Autodesk Inventor part; units mm, degrees
(part 2 of 3)
  line L933 (14.4439, 13.3712) -> (14.4659, 13.289)
  line L934 (14.4659, 13.289) -> (14.4484, 13.2234)
  line L935 (14.2154, 13.3626) -> (14.2397, 13.4369)
  line L936 (14.2397, 13.4369) -> (14.298, 13.5058)
  line L937 (14.298, 13.5058) -> (14.3807, 13.5279)
  line L938 (14.3807, 13.5279) -> (14.4634, 13.5058)
  line L939 (14.4634, 13.5058) -> (14.5239, 13.4453)
  line L940 (14.5239, 13.4453) -> (14.546, 13.3626)
  line L941 (14.546, 13.3626) -> (14.5239, 13.2799)
  line L942 (14.5239, 13.2799) -> (14.4484, 13.2234)
  line L943 (14.4484, 13.2234) -> (14.3807, 13.1972)
  line L944 (14.3807, 13.1972) -> (14.298, 13.2194)
  line L945 (14.298, 13.2194) -> (14.2375, 13.2799)
  line L946 (14.2375, 13.2799) -> (14.2154, 13.3626)
  line L947 (14.8734, 11.6652) -> (14.9343, 11.6816)
  line L948 (14.9343, 11.6816) -> (15.0165, 11.6595)
  line L949 (15.0165, 11.6595) -> (15.0767, 11.5993)
  line L950 (15.0767, 11.5993) -> (15.0987, 11.5171)
  line L951 (15.0987, 11.5171) -> (15.0767, 11.4349)
  line L952 (14.8517, 11.5809) -> (14.8734, 11.6652)
  line L953 (14.8734, 11.6652) -> (14.9343, 11.7241)
  line L954 (14.9343, 11.7241) -> (15.017, 11.7463)
  line L955 (15.017, 11.7463) -> (15.0997, 11.7241)
  line L956 (15.0997, 11.7241) -> (15.1602, 11.6636)
  line L957 (15.1602, 11.6636) -> (15.1823, 11.5809)
  line L958 (15.1823, 11.5809) -> (15.1602, 11.4982)
  line L959 (15.1602, 11.4982) -> (15.0997, 11.4377)
  line L960 (15.017, 11.4156) -> (14.9343, 11.4377)
  line L961 (14.9343, 11.4377) -> (14.8738, 11.4982)
  line L962 (14.8738, 11.4982) -> (14.8517, 11.5809)
  line L963 (14.8702, 9.3863) -> (14.9343, 9.4034)
  line L964 (14.9343, 9.4034) -> (15.0165, 9.3814)
  line L965 (15.0767, 9.1568) -> (15.0309, 9.111)
  line L966 (15.0165, 9.3814) -> (15.0767, 9.3212)
  line L967 (15.0767, 9.3212) -> (15.0987, 9.239)
  line L968 (15.0987, 9.239) -> (15.0767, 9.1568)
  line L969 (14.8517, 9.2902) -> (14.8702, 9.3863)
  line L970 (14.8702, 9.3863) -> (14.9343, 9.4334)
  line L971 (14.9343, 9.4334) -> (15.017, 9.4555)
  line L972 (15.017, 9.4555) -> (15.0997, 9.4334)
  line L973 (15.0997, 9.4334) -> (15.1602, 9.3729)
  line L974 (15.1602, 9.3729) -> (15.1823, 9.2902)
  line L975 (15.1823, 9.2902) -> (15.1602, 9.2075)
  line L976 (15.1602, 9.2075) -> (15.0997, 9.147)
  line L977 (15.0309, 9.111) -> (14.9343, 9.147)
  line L978 (14.9343, 9.147) -> (14.8738, 9.2075)
  line L979 (14.8738, 9.2075) -> (14.8517, 9.2902)
  line L980 (-2.5471, 11.8525) -> (-2.4869, 11.9127)
  line L981 (-2.5612, 11.9181) -> (-2.5007, 11.9786)
  line L982 (-2.1959, 13.1783) -> (-2.1357, 13.1181)
  line L983 (-2.2081, 13.2513) -> (-2.1475, 13.1907)
  line L984 (6.4547, 14.3394) -> (6.5369, 14.3173)
  line L985 (-16.6714, -15.6533) -> (-16.535, -15.1443)
  line L986 (-3.4172, 17.7096) -> (-3.0466, 17.339)
  line L987 (17.2697, -14.7625) -> (17.2918, -14.6798)
  line L988 (8.953, 17.2918) -> (8.8925, 17.3523)
  line L989 (8.8925, 17.3523) -> (8.8703, 17.435)
  line L990 (-2.3603, 13.1783) -> (-2.2781, 13.2003)
  line L991 (-2.3734, 13.2513) -> (-2.2907, 13.2734)
  line L992 (-4.4542, 16.0442) -> (-4.8268, 16.4169)
  line L993 (-2.1357, 13.1181) -> (-2.1475, 13.0254)
  line L994 (-2.2081, 12.9649) -> (-2.2907, 12.9427)
  line L995 (-2.4205, 13.1181) -> (-2.3603, 13.1783)
  line L996 (-2.4339, 13.1907) -> (-2.3734, 13.2513)
  line L997 (8.8925, 17.5177) -> (8.953, 17.5782)
  line L998 (8.9181, 14.1749) -> (8.9859, 13.9218)
  line L999 (16.0797, 11.6922) -> (16.0192, 11.7528)
  line L1000 (8.9859, 13.9218) -> (8.9277, 13.7046)
  line L1001 (8.4796, 14.4281) -> (8.7328, 14.3602)
  line L1002 (-2.1475, 13.1907) -> (-2.1357, 13.1181)
  line L1003 (-2.3067, 16.8433) -> (-2.3288, 16.9259)
  line L1004 (1.5431, 16.4996) -> (1.5652, 16.4169)
  line L1005 (8.2721, 14.4398) -> (8.5266, 14.508)
  line L1006 (8.0858, 14.2534) -> (8.2721, 14.4398)
  line L1007 (8.7811, 14.4398) -> (8.9675, 14.2534)
  line L1008 (16.0192, 11.7528) -> (15.997, 11.8354)
  line L1009 (8.5266, 14.508) -> (8.7811, 14.4398)
  line L1010 (-3.0634, 16.4169) -> (-3.4361, 16.0442)
  line L1011 (1.3999, 16.2516) -> (1.3172, 16.2737)
  line L1012 (-2.1475, 13.0254) -> (-2.2081, 12.9649)
  line L1013 (8.2265, 14.3602) -> (8.4796, 14.4281)
  line L1014 (8.0733, 14.207) -> (8.2265, 14.3602)
  line L1015 (9.0681, 17.4814) -> (9.1283, 17.4212)
  line L1016 (9.1183, 17.5782) -> (9.1788, 17.5177)
  line L1017 (8.7328, 14.3602) -> (8.9181, 14.1749)
  line L1018 (-3.4361, 16.0442) -> (-3.9451, 15.9078)
  line L1019 (-13.558, 10.4603) -> (-13.4978, 10.5205)
  line L1020 (8.9675, 14.2534) -> (9.0357, 13.9989)
  line L1021 (9.0357, 13.9989) -> (8.9675, 13.7444)
  line L1022 (8.7811, 13.5581) -> (8.5266, 13.4899)
  line L1023 (-14.8006, 2.418) -> (-14.7784, 2.5007)
  line L1024 (-3.9451, 15.9078) -> (-4.4542, 16.0442)
  line L1025 (8.5266, 13.4899) -> (8.2721, 13.5581)
  line L1026 (16.0192, 11.9181) -> (16.0797, 11.9786)
  line L1027 (1.4826, 16.2737) -> (1.3999, 16.2516)
  line L1028 (8.2721, 13.5581) -> (8.0858, 13.7444)
  line L1029 (1.4826, 16.5601) -> (1.5431, 16.4996)
  line L1030 (8.0858, 13.7444) -> (8.0176, 13.9989)
  line L1031 (8.9037, 17.4814) -> (8.9859, 17.5034)
  line L1032 (8.953, 17.5782) -> (9.0357, 17.6003)
  line L1033 (-2.2781, 13.2003) -> (-2.1959, 13.1783)
  line L1034 (-2.2907, 13.2734) -> (-2.2081, 13.2513)
  line L1035 (9.0357, 17.6003) -> (9.1183, 17.5782)
  line L1036 (16.2158, 11.8525) -> (16.2378, 11.7703)
  line L1037 (-4.9359, 16.8327) -> (-4.8003, 17.339)
  line L1038 (-3.9234, 17.8452) -> (-3.4172, 17.7096)
  line L1039 (-4.4297, 17.7096) -> (-3.9234, 17.8452)
  line L1040 (-4.8003, 17.339) -> (-4.4297, 17.7096)
  line L1041 (1.1391, 5.8597) -> (1.2213, 5.8377)
  line L1042 (1.0568, 5.8377) -> (1.1391, 5.8597)
  line L1043 (9.1503, 17.339) -> (9.1183, 17.2918)
  line L1044 (8.9859, 17.5034) -> (9.0681, 17.4814)
  line L1045 (8.8703, 17.435) -> (8.9037, 17.4814)
  line L1046 (-10.6691, 13.0359) -> (-10.647, 13.1181)
  line L1047 (-10.6497, 12.9637) -> (-10.6691, 13.0359)
  line L1048 (-10.5046, 13.2003) -> (-10.4229, 13.1784)
  line L1049 (-10.5868, 13.1783) -> (-10.5046, 13.2003)
  line L1050 (-10.647, 13.1181) -> (-10.5868, 13.1783)
  line L1051 (1.5346, 16.4087) -> (1.5538, 16.3371)
  line L1052 (1.4744, 16.4689) -> (1.5346, 16.4087)
  line L1053 (1.3922, 16.4909) -> (1.4744, 16.4689)
  line L1054 (1.31, 16.4689) -> (1.3922, 16.4909)
  line L1055 (1.2498, 16.4087) -> (1.31, 16.4689)
  line L1056 (-11.6816, 14.3015) -> (-11.6595, 14.3837)
  line L1057 (-11.6644, 14.2373) -> (-11.6816, 14.3015)
  line L1058 (-11.5171, 14.4659) -> (-11.4424, 14.4459)
  line L1059 (-11.5993, 14.4439) -> (-11.5171, 14.4659)
  line L1060 (-11.6595, 14.3837) -> (-11.5993, 14.4439)
  line L1061 (-13.58, 12.4031) -> (-13.558, 12.4853)
  line L1062 (-13.5609, 12.3317) -> (-13.58, 12.4031)
  line L1063 (-13.4156, 12.5675) -> (-13.348, 12.5494)
  line L1064 (-13.4978, 12.5455) -> (-13.4156, 12.5675)
  line L1065 (-13.558, 12.4853) -> (-13.4978, 12.5455)
  line L1066 (-14.5925, 11.3906) -> (-14.5705, 11.4728)
  line L1067 (-14.5723, 11.3154) -> (-14.5925, 11.3906)
  line L1068 (-14.4281, 11.555) -> (-14.3643, 11.5379)
  line L1069 (-14.5103, 11.533) -> (-14.4281, 11.555)
  line L1070 (-14.5705, 11.4728) -> (-14.5103, 11.533)
  line L1071 (-8.391, 17.339) -> (-8.3689, 17.4212)
  line L1072 (-8.1443, 17.4814) -> (-8.1023, 17.4394)
  line L1073 (-8.2265, 17.5034) -> (-8.1443, 17.4814)
  line L1074 (-8.3087, 17.4814) -> (-8.2265, 17.5034)
  line L1075 (-8.3689, 17.4212) -> (-8.3087, 17.4814)
  line L1076 (-7.1232, 17.3471) -> (-7.1033, 17.4212)
  line L1077 (-6.8787, 17.4814) -> (-6.8332, 17.4359)
  line L1078 (-6.9609, 17.5034) -> (-6.8787, 17.4814)
  line L1079 (-7.0431, 17.4814) -> (-6.9609, 17.5034)
  line L1080 (-7.1033, 17.4212) -> (-7.0431, 17.4814)
  line L1081 (-17.5034, 5.9484) -> (-17.4814, 6.0306)
  line L1082 (-17.4814, 5.8662) -> (-17.5034, 5.9484)
  line L1083 (-17.4331, 5.8179) -> (-17.4814, 5.8662)
  line L1084 (-17.4212, 6.0908) -> (-17.3485, 6.1103)
  line L1085 (-17.4814, 6.0306) -> (-17.4212, 6.0908)
  line L1086 (-17.5034, 0.8859) -> (-17.4814, 0.9681)
  line L1087 (-17.4814, 0.8037) -> (-17.5034, 0.8859)
  line L1088 (-17.4212, 0.7435) -> (-17.4814, 0.8037)
  line L1089 (-17.3944, 0.7364) -> (-17.4212, 0.7435)
  line L1090 (-17.4212, 1.0283) -> (-17.3555, 1.0459)
  line L1091 (-17.4814, 0.9681) -> (-17.4212, 1.0283)
  line L1092 (-14.3394, -4.4297) -> (-14.3173, -4.3474)
  line L1093 (-14.3173, -4.5119) -> (-14.3394, -4.4297)
  line L1094 (-14.2571, -4.5721) -> (-14.3173, -4.5119)
  line L1095 (-14.1749, -4.5941) -> (-14.2571, -4.5721)
  line L1096 (-14.3173, -4.3474) -> (-14.2571, -4.2873)
  line L1097 (-17.3768, -10.5046) -> (-17.3548, -10.4224)
  line L1098 (-17.3548, -10.5868) -> (-17.3768, -10.5046)
  line L1099 (-17.2946, -10.647) -> (-17.3548, -10.5868)
  line L1100 (-17.2124, -10.6691) -> (-17.2946, -10.647)
  line L1101 (-17.1619, -10.6555) -> (-17.2124, -10.6691)
  line L1102 (-17.3548, -10.4224) -> (-17.3188, -10.3864)
  line L1103 (-14.4659, -12.5296) -> (-14.4473, -12.4601)
  line L1104 (-14.4439, -12.6118) -> (-14.4659, -12.5296)
  line L1105 (-14.3837, -12.672) -> (-14.4439, -12.6118)
  line L1106 (-14.3015, -12.6941) -> (-14.3837, -12.672)
  line L1107 (-14.2387, -12.6772) -> (-14.3015, -12.6941)
  line L1108 (-15.7315, -6.9609) -> (-15.7095, -6.8787)
  line L1109 (-15.7095, -7.0431) -> (-15.7315, -6.9609)
  line L1110 (-15.6493, -7.1033) -> (-15.7095, -7.0431)
  line L1111 (-15.5671, -7.1253) -> (-15.6493, -7.1033)
  line L1112 (-15.7095, -6.8787) -> (-15.6591, -6.8283)
  line L1113 (-14.4659, -10.7578) -> (-14.4448, -10.6791)
  line L1114 (-14.4439, -10.84) -> (-14.4659, -10.7578)
  line L1115 (-14.3837, -10.9002) -> (-14.4439, -10.84)
  line L1116 (-14.3015, -10.9222) -> (-14.3837, -10.9002)
  line L1117 (-14.2362, -10.9047) -> (-14.3015, -10.9222)
  line L1118 (-16.9972, -12.0234) -> (-16.9751, -11.9412)
  line L1119 (-16.9751, -12.1056) -> (-16.9972, -12.0234)
  line L1120 (-16.9149, -12.1658) -> (-16.9751, -12.1056)
  line L1121 (-16.8327, -12.1878) -> (-16.9149, -12.1658)
  line L1122 (-16.7823, -12.1743) -> (-16.8327, -12.1878)
  line L1123 (-17.2503, -13.5421) -> (-17.2296, -13.4649)
  line L1124 (-17.2283, -13.6243) -> (-17.2503, -13.5421)
  line L1125 (-17.1681, -13.6845) -> (-17.2283, -13.6243)
  line L1126 (-17.0859, -13.7065) -> (-17.1681, -13.6845)
  line L1127 (-17.0388, -13.694) -> (-17.0859, -13.7065)
  line L1128 (-11.1753, -15.314) -> (-11.1593, -15.2543)
  line L1129 (-11.1533, -15.3962) -> (-11.1753, -15.314)
  line L1130 (-11.0931, -15.4564) -> (-11.1533, -15.3962)
  line L1131 (-11.0109, -15.4784) -> (-11.0931, -15.4564)
  line L1132 (-10.9287, -15.4564) -> (-11.0109, -15.4784)
  line L1133 (-8.8972, -17.339) -> (-8.8832, -17.2866)
  line L1134 (-8.8752, -17.4212) -> (-8.8972, -17.339)
  line L1135 (-8.815, -17.4814) -> (-8.8752, -17.4212)
  line L1136 (-8.7328, -17.5034) -> (-8.815, -17.4814)
  line L1137 (-8.6506, -17.4814) -> (-8.7328, -17.5034)
  line L1138 (-8.61, -17.4408) -> (-8.6506, -17.4814)
  line L1139 (-6.5971, -17.4212) -> (-6.6167, -17.3478)
  line L1140 (-6.5369, -17.4814) -> (-6.5971, -17.4212)
  line L1141 (-6.4547, -17.5034) -> (-6.5369, -17.4814)
  line L1142 (-6.3724, -17.4814) -> (-6.4547, -17.5034)
  line L1143 (-6.3256, -17.4345) -> (-6.3724, -17.4814)
  line L1144 (-0.0158, -17.4212) -> (-0.0331, -17.3569)
  line L1145 (0.0443, -17.4814) -> (-0.0158, -17.4212)
  line L1146 (0.1266, -17.5034) -> (0.0443, -17.4814)
  line L1147 (0.2088, -17.4814) -> (0.1266, -17.5034)
  line L1148 (0.2863, -17.3566) -> (0.269, -17.4212)
  line L1149 (5.8662, -15.7095) -> (5.813, -15.6563)
  line L1150 (5.9484, -15.7315) -> (5.8662, -15.7095)
  line L1151 (6.0306, -15.7095) -> (5.9484, -15.7315)
  line L1152 (6.0908, -15.6493) -> (6.0306, -15.7095)
  line L1153 (6.1127, -15.5675) -> (6.0908, -15.6493)
  line L1154 (8.9037, -14.9501) -> (8.8568, -14.9033)
  line L1155 (8.9859, -14.9722) -> (8.9037, -14.9501)
  line L1156 (9.0681, -14.9501) -> (8.9859, -14.9722)
  line L1157 (9.1283, -14.89) -> (9.0681, -14.9501)
  line L1158 (9.1503, -14.8077) -> (9.1283, -14.89)
  line L1159 (9.1329, -14.7427) -> (9.1503, -14.8077)
  line L1160 (11.7703, -14.9722) -> (11.6975, -14.9527)
  line L1161 (11.8525, -14.9501) -> (11.7703, -14.9722)
  line L1162 (11.9127, -14.89) -> (11.8525, -14.9501)
  line L1163 (11.9347, -14.8077) -> (11.9127, -14.89)
  line L1164 (11.9183, -14.7465) -> (11.9347, -14.8077)
  line L1165 (13.5421, -15.9847) -> (13.467, -15.9645)
  line L1166 (13.6243, -15.9626) -> (13.5421, -15.9847)
  line L1167 (13.6845, -15.9024) -> (13.6243, -15.9626)
  line L1168 (13.7065, -15.8202) -> (13.6845, -15.9024)
  line L1169 (13.6922, -15.7667) -> (13.7065, -15.8202)
  line L1170 (15.0609, -17.3768) -> (14.9925, -17.3585)
  line L1171 (15.1431, -17.3548) -> (15.0609, -17.3768)
  line L1172 (15.2033, -17.2946) -> (15.1431, -17.3548)
  line L1173 (15.2253, -17.2124) -> (15.2033, -17.2946)
  line L1174 (15.2134, -17.1682) -> (15.2253, -17.2124)
  line L1175 (17.339, -14.8456) -> (17.2949, -14.8338)
  line L1176 (17.4212, -14.8236) -> (17.339, -14.8456)
  line L1177 (17.4814, -14.7634) -> (17.4212, -14.8236)
  line L1178 (17.5034, -14.6812) -> (17.4814, -14.7634)
  line L1179 (17.4844, -14.6104) -> (17.5034, -14.6812)
  line L1180 (15.5671, -13.4534) -> (15.5119, -13.4386)
  line L1181 (15.6493, -13.4314) -> (15.5671, -13.4534)
  line L1182 (15.7095, -13.3712) -> (15.6493, -13.4314)
  line L1183 (15.7315, -13.289) -> (15.7095, -13.3712)
  line L1184 (15.7111, -13.2127) -> (15.7315, -13.289)
  line L1185 (17.4814, 9.1568) -> (17.4422, 9.1176)
  line L1186 (17.5034, 9.239) -> (17.4814, 9.1568)
  line L1187 (17.4814, 9.3212) -> (17.5034, 9.239)
  line L1188 (17.4212, 9.3814) -> (17.4814, 9.3212)
  line L1189 (17.339, 9.4034) -> (17.4212, 9.3814)
  line L1190 (17.2873, 9.3896) -> (17.339, 9.4034)
  line L1191 (17.4814, 11.4349) -> (17.4485, 11.4021)
  line L1192 (17.5034, 11.5171) -> (17.4814, 11.4349)
  line L1193 (17.4814, 11.5993) -> (17.5034, 11.5171)
  line L1194 (17.4212, 11.6595) -> (17.4814, 11.5993)
  line L1195 (17.339, 11.6816) -> (17.4212, 11.6595)
  line L1196 (17.2905, 11.6686) -> (17.339, 11.6816)
  line L1197 (17.2503, 12.7827) -> (17.2284, 12.701)
  line L1198 (17.2283, 12.865) -> (17.2503, 12.7827)
  line L1199 (17.1681, 12.9251) -> (17.2283, 12.865)
  line L1200 (17.0859, 12.9472) -> (17.1681, 12.9251)
  line L1201 (17.0373, 12.9362) -> (17.0859, 12.9472)
  line L1202 (15.9847, 13.0359) -> (15.9637, 12.9577)
  line L1203 (14.2128, 17.339) -> (14.2007, 17.294)
  line L1204 (14.1908, 17.4212) -> (14.2128, 17.339)
  line L1205 (14.1306, 17.4814) -> (14.1908, 17.4212)
  line L1206 (14.0484, 17.5034) -> (14.1306, 17.4814)
  line L1207 (13.9738, 17.4834) -> (14.0484, 17.5034)
  line L1208 (12.9472, 17.339) -> (12.9347, 17.2922)
  line L1209 (12.9251, 17.4212) -> (12.9472, 17.339)
  line L1210 (12.865, 17.4814) -> (12.9251, 17.4212)
  line L1211 (12.7827, 17.5034) -> (12.865, 17.4814)
  line L1212 (12.7006, 17.4814) -> (12.7827, 17.5034)
  line L1213 (10.9222, 17.339) -> (10.9089, 17.2894)
  line L1214 (16.2378, 11.7703) -> (16.2158, 11.688)
  line L1215 (16.1556, 11.9127) -> (16.2158, 11.8525)
  line L1216 (16.0192, 11.9181) -> (16.0734, 11.9347)
  line L1217 (6.5971, 14.2571) -> (6.6191, 14.1749)
  line L1218 (6.5369, 14.3173) -> (6.5971, 14.2571)
  line L1219 (5.5846, 14.004) -> (5.6155, 13.9162)
  line L1220 (5.5244, 14.0642) -> (5.5846, 14.004)
  line L1221 (5.4422, 14.0862) -> (5.5244, 14.0642)
  line L1222 (5.3599, 14.0642) -> (5.4422, 14.0862)
  line L1223 (-5.8662, 16.4689) -> (-5.8151, 16.4178)
  line L1224 (-5.9484, 16.4909) -> (-5.8662, 16.4689)
  line L1225 (-6.0306, 16.4689) -> (-5.9484, 16.4909)
  line L1226 (-6.0908, 16.4087) -> (-6.0306, 16.4689)
  line L1227 (-6.1128, 15.0609) -> (-6.0908, 15.1431)
  line L1228 (-5.8662, 15.2033) -> (-5.8116, 15.1487)
  line L1229 (-5.9484, 15.2253) -> (-5.8662, 15.2033)
  line L1230 (-6.0306, 15.2033) -> (-5.9484, 15.2253)
  line L1231 (-6.0908, 15.1431) -> (-6.0306, 15.2033)
  line L1232 (-4.3409, 15.0611) -> (-4.3189, 15.1431)
  line L1233 (-4.0943, 15.2033) -> (-4.0348, 15.1438)
  line L1234 (-4.1765, 15.2253) -> (-4.0943, 15.2033)
  line L1235 (-4.2588, 15.2033) -> (-4.1765, 15.2253)
  line L1236 (-4.3189, 15.1431) -> (-4.2588, 15.2033)
  line L1237 (-12.4031, 11.555) -> (-12.3286, 11.5363)
  line L1238 (-12.4853, 11.533) -> (-12.4031, 11.555)
  line L1239 (-15.4784, 10.5046) -> (-15.4564, 10.5868)
  line L1240 (-15.4564, 10.4224) -> (-15.4784, 10.5046)
  line L1241 (-15.314, 10.6691) -> (-15.2536, 10.6529)
  line L1242 (-15.3962, 10.647) -> (-15.314, 10.6691)
  line L1243 (-15.4564, 10.5868) -> (-15.3962, 10.647)
  line L1244 (-2.3067, 16.8433) -> (-2.294, 16.9149)
  line L1245 (-2.0693, 16.9751) -> (-2.0092, 16.9149)
  line L1246 (-2.1516, 16.9972) -> (-2.0693, 16.9751)
  line L1247 (-2.2338, 16.9751) -> (-2.1516, 16.9972)
  line L1248 (-2.294, 16.9149) -> (-2.2338, 16.9751)
  line L1249 (-13.58, 10.3781) -> (-13.558, 10.4603)
  line L1250 (-13.5581, 10.2962) -> (-13.58, 10.3781)
  line L1251 (-13.4978, 10.5205) -> (-13.4156, 10.5425)
  line L1252 (-14.2128, 3.6703) -> (-14.1908, 3.7525)
  line L1253 (-14.1908, 3.5881) -> (-14.2128, 3.6703)
  line L1254 (-14.1306, 3.5279) -> (-14.1908, 3.5881)
  line L1255 (-14.1306, 3.8127) -> (-14.0484, 3.8347)
  line L1256 (-14.1908, 3.7525) -> (-14.1306, 3.8127)
  line L1257 (-17.4814, -0.8416) -> (-17.5034, -0.7594)
  line L1258 (-17.4212, -0.9018) -> (-17.4814, -0.8416)
  line L1259 (-17.3557, -0.9193) -> (-17.4212, -0.9018)
  line L1260 (-16.2378, -0.6328) -> (-16.2158, -0.5506)
  line L1261 (-16.2158, -0.715) -> (-16.2378, -0.6328)
  line L1262 (-16.1556, -0.7752) -> (-16.2158, -0.715)
  line L1263 (-16.0837, -0.7945) -> (-16.1556, -0.7752)
  line L1264 (-16.2158, -0.5506) -> (-16.1556, -0.4904)
  line L1265 (-15.0987, -5.6953) -> (-15.0767, -5.6131)
  line L1266 (-15.0767, -5.7775) -> (-15.0987, -5.6953)
  line L1267 (-15.0165, -5.8377) -> (-15.0767, -5.7775)
  line L1268 (-14.9343, -5.8597) -> (-15.0165, -5.8377)
  line L1269 (-15.0767, -5.6131) -> (-15.0211, -5.5574)
  line L1270 (-13.7065, -5.9484) -> (-13.6845, -5.8662)
  line L1271 (-13.6845, -6.0306) -> (-13.7065, -5.9484)
  line L1272 (-13.6243, -6.0908) -> (-13.6845, -6.0306)
  line L1273 (-13.5421, -6.1128) -> (-13.6243, -6.0908)
  line L1274 (-13.6845, -5.8662) -> (-13.6257, -5.8074)
  line L1275 (-14.2128, -7.9734) -> (-14.1908, -7.8912)
  line L1276 (-14.1908, -8.0556) -> (-14.2128, -7.9734)
  line L1277 (-14.1306, -8.1158) -> (-14.1908, -8.0556)
  line L1278 (-14.0484, -8.1378) -> (-14.1306, -8.1158)
  line L1279 (-13.978, -8.119) -> (-14.0484, -8.1378)
  line L1280 (-14.1908, -7.8912) -> (-14.139, -7.8394)
  line L1281 (-12.4409, -12.2765) -> (-12.4212, -12.2029)
  line L1282 (-12.4189, -12.3587) -> (-12.4409, -12.2765)
  line L1283 (-12.3587, -12.4189) -> (-12.4189, -12.3587)
  line L1284 (-12.2765, -12.4409) -> (-12.3587, -12.4189)
  line L1285 (-12.2029, -12.4212) -> (-12.2765, -12.4409)
  line L1286 (-8.7706, -13.7952) -> (-8.7517, -13.7244)
  line L1287 (-8.7486, -13.8775) -> (-8.7706, -13.7952)
  line L1288 (-8.6884, -13.9376) -> (-8.7486, -13.8775)
  line L1289 (-8.6062, -13.9597) -> (-8.6884, -13.9376)
  line L1290 (-8.524, -13.9376) -> (-8.6062, -13.9597)
  line L1291 (-8.4997, -13.9134) -> (-8.524, -13.9376)
  line L1292 (0.8037, -15.4564) -> (0.7435, -15.3962)
  line L1293 (0.8859, -15.4784) -> (0.8037, -15.4564)
  line L1294 (0.9681, -15.4564) -> (0.8859, -15.4784)
  line L1295 (1.0283, -15.3962) -> (0.9681, -15.4564)
  line L1296 (1.0487, -15.3201) -> (1.0283, -15.3962)
  line L1297 (13.558, -13.4978) -> (13.4978, -13.558)
  line L1298 (13.58, -13.4156) -> (13.558, -13.4978)
  line L1299 (13.5623, -13.3494) -> (13.58, -13.4156)
  line L1300 (13.3269, 10.5046) -> (13.305, 10.4231)
  line L1301 (13.3048, 10.5868) -> (13.3269, 10.5046)
  line L1302 (13.2446, 10.647) -> (13.3048, 10.5868)
  line L1303 (13.1624, 10.6691) -> (13.2446, 10.647)
  line L1304 (13.0909, 10.6499) -> (13.1624, 10.6691)
  line L1305 (11.1832, 12.9362) -> (11.264, 12.9472)
  line L1306 (-17.5034, 4.05) -> (-17.4814, 4.1322)
  line L1307 (-17.4814, 3.9678) -> (-17.5034, 4.05)
  line L1308 (-17.4278, 3.9142) -> (-17.4814, 3.9678)
  line L1309 (-17.4212, 4.1924) -> (-17.3511, 4.2112)
  line L1310 (-17.4814, 4.1322) -> (-17.4212, 4.1924)
  line L1311 (-17.5034, 2.5312) -> (-17.4814, 2.6135)
  line L1312 (-17.4236, 2.3913) -> (-17.4814, 2.449)
  line L1313 (-17.4212, 2.6736) -> (-17.3532, 2.6918)
  line L1314 (-17.4814, 2.6135) -> (-17.4212, 2.6736)
  line L1315 (-5.2049, -0.0822) -> (-5.2269, 0)
  line L1316 (-5.1447, -0.1424) -> (-5.2049, -0.0822)
  line L1317 (1.5346, 12.2322) -> (1.5566, 12.1499)
  line L1318 (1.4744, 12.2923) -> (1.5346, 12.2322)
  line L1319 (1.3922, 12.3144) -> (1.4744, 12.2923)
  line L1320 (1.31, 12.2923) -> (1.3922, 12.3144)
  line L1321 (1.2498, 12.2322) -> (1.31, 12.2923)
  line L1322 (-3.455, 12.6562) -> (-3.433, 12.7384)
  line L1323 (-3.2084, 12.7986) -> (-3.1482, 12.7384)
  line L1324 (-3.2906, 12.8206) -> (-3.2084, 12.7986)
  line L1325 (-3.3728, 12.7986) -> (-3.2906, 12.8206)
  line L1326 (-3.433, 12.7384) -> (-3.3728, 12.7986)
  line L1327 (-2.5691, 11.7703) -> (-2.5471, 11.8525)
  line L1328 (-2.3225, 11.9127) -> (-2.2623, 11.8525)
  line L1329 (-2.4047, 11.9347) -> (-2.3225, 11.9127)
  line L1330 (-2.4869, 11.9127) -> (-2.4047, 11.9347)
  line L1331 (-1.3035, 13.0359) -> (-1.2815, 13.1181)
  line L1332 (-1.0568, 13.1783) -> (-0.9967, 13.1181)
  line L1333 (-1.1391, 13.2003) -> (-1.0568, 13.1783)
  line L1334 (-1.2213, 13.1783) -> (-1.1391, 13.2003)
  line L1335 (-1.2815, 13.1181) -> (-1.2213, 13.1783)
  line L1336 (4.4455, 12.9915) -> (4.4675, 12.9093)
  line L1337 (4.3853, 13.0517) -> (4.4455, 12.9915)
  line L1338 (4.3031, 13.0737) -> (4.3853, 13.0517)
  line L1339 (4.2209, 13.0517) -> (4.3031, 13.0737)
  line L1340 (4.1607, 12.9915) -> (4.2209, 13.0517)
  line L1341 (-3.7525, -2.294) -> (-3.8127, -2.2338)
  line L1342 (1.4744, 8.622) -> (1.5346, 8.5619)
  line L1343 (1.3922, 8.6441) -> (1.4744, 8.622)
  line L1344 (1.31, 8.622) -> (1.3922, 8.6441)
  line L1345 (1.2498, 8.5619) -> (1.31, 8.622)
  line L1346 (15.0767, 4.6006) -> (15.0183, 4.5421)
  line L1347 (15.0987, 4.6828) -> (15.0767, 4.6006)
  line L1348 (15.0767, 4.765) -> (15.0987, 4.6828)
  line L1349 (15.0165, 4.8252) -> (15.0767, 4.765)
  line L1350 (14.9343, 4.8472) -> (15.0165, 4.8252)
  line L1351 (15.3962, -0.7752) -> (15.3161, -0.7795)
  line L1352 (15.4564, -0.715) -> (15.3962, -0.7752)
  line L1353 (15.4784, -0.6328) -> (15.4564, -0.715)
  line L1354 (15.4564, -0.5506) -> (15.4784, -0.6328)
  line L1355 (15.3988, -0.471) -> (15.4564, -0.5506)
  line L1356 (-13.4534, 2.1516) -> (-13.4314, 2.2338)
  line L1357 (-13.4314, 2.0693) -> (-13.4534, 2.1516)
  line L1358 (-13.3712, 2.0092) -> (-13.4314, 2.0693)
  line L1359 (-13.3712, 2.294) -> (-13.289, 2.316)
  line L1360 (-13.4314, 2.2338) -> (-13.3712, 2.294)
  line L1361 (-14.719, 2.4047) -> (-14.697, 2.4869)
  line L1362 (-14.697, 2.3225) -> (-14.719, 2.4047)
  line L1363 (-14.6368, 2.2623) -> (-14.697, 2.3225)
  line L1364 (-14.6368, 2.5471) -> (-14.5547, 2.5691)
  line L1365 (-14.697, 2.4869) -> (-14.6368, 2.5471)
  line L1366 (-11.1753, -2.1516) -> (-11.1533, -2.0693)
  line L1367 (-11.1533, -2.2338) -> (-11.1753, -2.1516)
  line L1368 (-11.0931, -2.294) -> (-11.1533, -2.2338)
  line L1369 (-11.0109, -2.316) -> (-11.0931, -2.294)
  line L1370 (-11.1533, -2.0693) -> (-11.0931, -2.0092)
  line L1371 (-16.9751, 7.0052) -> (-16.9972, 7.0875)
  line L1372 (-16.9286, 6.9587) -> (-16.9751, 7.0052)
  line L1373 (-16.9149, 7.2299) -> (-16.8381, 7.2505)
  line L1374 (-16.9751, 7.1697) -> (-16.9149, 7.2299)
  line L1375 (-7.9734, 7.7203) -> (-7.9395, 7.8468)
  line L1376 (-7.9395, 7.5937) -> (-7.9734, 7.7203)
  line L1377 (-7.7203, 7.9734) -> (-7.5937, 7.9395)
  line L1378 (-7.8468, 7.9395) -> (-7.7203, 7.9734)
  line L1379 (-7.9395, 7.8468) -> (-7.8468, 7.9395)
  line L1380 (7.9734, 7.7203) -> (7.9395, 7.5937)
  line L1381 (7.9395, 7.8468) -> (7.9734, 7.7203)
  line L1382 (7.8468, 7.9395) -> (7.9395, 7.8468)
  line L1383 (7.7203, 7.9734) -> (7.8468, 7.9395)
  line L1384 (7.5937, 7.9395) -> (7.7203, 7.9734)
  line L1385 (-7.9395, -7.8468) -> (-7.9734, -7.7203)
  line L1386 (-7.8468, -7.9395) -> (-7.9395, -7.8468)
  line L1387 (-7.5937, -7.9395) -> (-7.7203, -7.9734)
  line L1388 (7.7203, -7.9734) -> (7.5937, -7.9395)
  line L1389 (7.8468, -7.9395) -> (7.7203, -7.9734)
  line L1390 (7.9734, -7.7203) -> (7.9395, -7.8468)
  line L1391 (16.3056, 11.9181) -> (16.3277, 11.8354)
  line L1392 (-15.6533, -14.6352) -> (-15.1443, -14.7716)
  line L1393 (-15.1443, -14.7716) -> (-14.7716, -15.1443)
  line L1394 (-14.7716, -15.1443) -> (-14.6352, -15.6533)
  line L1395 (-14.6352, -15.6533) -> (-14.7716, -16.1624)
  line L1396 (-15.1443, -16.535) -> (-15.6533, -16.6714)
  line L1397 (-15.6533, -16.6714) -> (-16.1624, -16.535)
  line L1398 (-16.1624, -16.535) -> (-16.535, -16.1624)
  line L1399 (-16.535, -16.1624) -> (-16.6714, -15.6533)
  line L1400 (-4.9632, 16.9259) -> (-4.8268, 17.435)
  line L1401 (-4.8268, 17.435) -> (-4.4542, 17.8076)
  line L1402 (-4.4542, 17.8076) -> (-3.9451, 17.944)
  line L1403 (-3.9451, 17.944) -> (-3.4361, 17.8076)
  line L1404 (-3.4361, 17.8076) -> (-3.0634, 17.435)
  line L1405 (-2.927, 16.9259) -> (-3.0634, 16.4169)
  line L1406 (0.98, 5.7268) -> (1.0022, 5.8095)
  line L1407 (1.0627, 5.87) -> (1.1454, 5.8922)
  line L1408 (1.1454, 5.8922) -> (1.228, 5.87)
  line L1409 (1.228, 5.87) -> (1.2886, 5.8095)
  line L1410 (1.2886, 5.6442) -> (1.228, 5.5836)
  line L1411 (1.228, 5.5836) -> (1.1454, 5.5615)
  line L1412 (1.1454, 5.5615) -> (1.0627, 5.5836)
  line L1413 (1.0627, 5.5836) -> (1.0022, 5.6442)
  line L1414 (1.0022, 5.6442) -> (0.98, 5.7268)
  line L1415 (-2.2907, 12.9427) -> (-2.3734, 12.9649)
  line L1416 (-2.3734, 12.9649) -> (-2.4425, 13.0359)
  line L1417 (-2.4425, 13.0359) -> (-2.4561, 13.1081)
  line L1418 (9.201, 17.435) -> (9.1788, 17.3523)
  line L1419 (9.1183, 17.2918) -> (9.0357, 17.2697)
  line L1420 (11.6922, 17.5177) -> (11.7528, 17.5782)
  line L1421 (11.7528, 17.5782) -> (11.8354, 17.6003)
  line L1422 (11.8354, 17.6003) -> (11.9181, 17.5782)
  line L1423 (11.9181, 17.5782) -> (11.9786, 17.5177)
  line L1424 (11.9786, 17.5177) -> (12.0008, 17.435)
  line L1425 (12.0008, 17.435) -> (11.9786, 17.3523)
  line L1426 (11.9786, 17.3523) -> (11.9218, 17.2908)
  line L1427 (11.9218, 17.2908) -> (11.8354, 17.2697)
  line L1428 (11.8354, 17.2697) -> (11.7528, 17.2918)
  line L1429 (11.7528, 17.2918) -> (11.6922, 17.3523)
  line L1430 (11.6922, 17.3523) -> (11.6559, 17.4492)
  line L1431 (-10.7282, 13.1081) -> (-10.706, 13.1907)
  line L1432 (-10.706, 13.1907) -> (-10.6455, 13.2513)
  line L1433 (-10.6455, 13.2513) -> (-10.5628, 13.2734)
  line L1434 (-10.5628, 13.2734) -> (-10.4801, 13.2513)
  line L1435 (-10.4801, 13.2513) -> (-10.4229, 13.1784)
  line L1436 (-10.4229, 13.1784) -> (-10.3975, 13.1081)
  line L1437 (-10.3975, 13.1081) -> (-10.4196, 13.0254)
  line L1438 (-10.4196, 13.0254) -> (-10.4801, 12.9649)
  line L1439 (-10.4801, 12.9649) -> (-10.5628, 12.9427)
  line L1440 (-10.5628, 12.9427) -> (-10.6497, 12.9637)
  line L1441 (-10.6497, 12.9637) -> (-10.706, 13.0254)
  line L1442 (-10.706, 13.0254) -> (-10.7282, 13.1081)
  line L1443 (1.2498, 16.4087) -> (1.2567, 16.4996)
  line L1444 (1.3172, 16.5601) -> (1.3999, 16.5822)
  line L1445 (1.5652, 16.4169) -> (1.5538, 16.3371)
  line L1446 (1.5538, 16.3371) -> (1.4826, 16.2737)
  line L1447 (1.3172, 16.2737) -> (1.2567, 16.3342)
  line L1448 (1.2567, 16.3342) -> (1.2498, 16.4087)
  line L1449 (-11.7463, 14.3807) -> (-11.7241, 14.4634)
  line L1450 (-11.7241, 14.4634) -> (-11.6636, 14.5239)
  line L1451 (-11.6636, 14.5239) -> (-11.5809, 14.546)
  line L1452 (-11.5809, 14.546) -> (-11.4982, 14.5239)
  line L1453 (-11.4982, 14.5239) -> (-11.4424, 14.4459)
  line L1454 (-11.4424, 14.4459) -> (-11.4156, 14.3807)
  line L1455 (-11.4156, 14.3807) -> (-11.4377, 14.298)
  line L1456 (-11.4377, 14.298) -> (-11.4982, 14.2375)
  line L1457 (-11.4982, 14.2375) -> (-11.5809, 14.2154)
  line L1458 (-11.5809, 14.2154) -> (-11.6644, 14.2373)
  line L1459 (-11.6644, 14.2373) -> (-11.7241, 14.298)
  line L1460 (-11.7241, 14.298) -> (-11.7463, 14.3807)
  line L1461 (-13.6552, 12.4718) -> (-13.633, 12.5544)
  line L1462 (-13.633, 12.5544) -> (-13.5725, 12.6149)
  line L1463 (-13.5725, 12.6149) -> (-13.4899, 12.6371)
  line L1464 (-13.4899, 12.6371) -> (-13.4072, 12.6149)
  line L1465 (-13.4072, 12.6149) -> (-13.348, 12.5494)
  line L1466 (-13.348, 12.5494) -> (-13.3245, 12.4718)
  line L1467 (-13.3245, 12.4718) -> (-13.3467, 12.3891)
  line L1468 (-13.3467, 12.3891) -> (-13.4072, 12.3286)
  line L1469 (-13.4072, 12.3286) -> (-13.4899, 12.3064)
  line L1470 (-13.4899, 12.3064) -> (-13.5609, 12.3317)
  line L1471 (-13.5609, 12.3317) -> (-13.633, 12.3891)
  line L1472 (-13.633, 12.3891) -> (-13.6552, 12.4718)
  line L1473 (-14.6733, 11.4536) -> (-14.6511, 11.5363)
  line L1474 (-14.6511, 11.5363) -> (-14.5906, 11.5968)
  line L1475 (-14.5906, 11.5968) -> (-14.508, 11.619)
  line L1476 (-14.508, 11.619) -> (-14.4253, 11.5968)
  line L1477 (-14.4253, 11.5968) -> (-14.3643, 11.5379)
  line L1478 (-14.3643, 11.5379) -> (-14.3426, 11.4536)
  line L1479 (-14.3426, 11.4536) -> (-14.3648, 11.371)
  line L1480 (-14.3648, 11.371) -> (-14.4253, 11.3105)
  line L1481 (-14.4253, 11.3105) -> (-14.508, 11.2883)
  line L1482 (-14.508, 11.2883) -> (-14.5723, 11.3154)
  line L1483 (-14.5723, 11.3154) -> (-14.6511, 11.371)
  line L1484 (-14.6511, 11.371) -> (-14.6733, 11.4536)
  line L1485 (-8.4374, 17.435) -> (-8.4153, 17.5177)
  line L1486 (-8.4153, 17.5177) -> (-8.3547, 17.5782)
  line L1487 (-8.3547, 17.5782) -> (-8.2721, 17.6003)
  line L1488 (-8.2721, 17.6003) -> (-8.1894, 17.5782)
  line L1489 (-8.1894, 17.5782) -> (-8.1289, 17.5177)
  line L1490 (-8.1289, 17.5177) -> (-8.1023, 17.4394)
  line L1491 (-8.1023, 17.4394) -> (-8.1289, 17.3523)
  line L1492 (-8.1289, 17.3523) -> (-8.1894, 17.2918)
  line L1493 (-8.1894, 17.2918) -> (-8.2721, 17.2697)
  line L1494 (-8.2721, 17.2697) -> (-8.3547, 17.2918)
  line L1495 (-8.4153, 17.3523) -> (-8.4374, 17.435)
  line L1496 (-6.0194, 17.435) -> (-5.9973, 17.5177)
  line L1497 (-5.9973, 17.5177) -> (-5.9368, 17.5782)
  line L1498 (-5.9368, 17.5782) -> (-5.8541, 17.6003)
  line L1499 (-5.8541, 17.6003) -> (-5.7714, 17.5782)
  line L1500 (-5.7714, 17.5782) -> (-5.7109, 17.5177)
  line L1501 (-5.7109, 17.5177) -> (-5.691, 17.4327)
  line L1502 (-5.691, 17.4327) -> (-5.7109, 17.3523)
  line L1503 (-5.7109, 17.3523) -> (-5.7714, 17.2918)
  line L1504 (-5.7714, 17.2918) -> (-5.8541, 17.2697)
  line L1505 (-5.8541, 17.2697) -> (-5.9368, 17.2918)
  line L1506 (-5.9368, 17.2918) -> (-5.9837, 17.3487)
  line L1507 (-5.9837, 17.3487) -> (-6.0194, 17.435)
  line L1508 (-7.1648, 17.435) -> (-7.1426, 17.5177)
  line L1509 (-7.1426, 17.5177) -> (-7.0821, 17.5782)
  line L1510 (-7.0821, 17.5782) -> (-6.9995, 17.6003)
  line L1511 (-6.9995, 17.6003) -> (-6.9168, 17.5782)
  line L1512 (-6.9168, 17.5782) -> (-6.8563, 17.5177)
  line L1513 (-6.8563, 17.5177) -> (-6.8332, 17.4359)
  line L1514 (-6.8332, 17.4359) -> (-6.8563, 17.3523)
  line L1515 (-6.8563, 17.3523) -> (-6.9168, 17.2918)
  line L1516 (-6.9168, 17.2918) -> (-6.9995, 17.2697)
  line L1517 (-6.9995, 17.2697) -> (-7.0821, 17.2918)
  line L1518 (-7.0821, 17.2918) -> (-7.1232, 17.3471)
  line L1519 (-7.1232, 17.3471) -> (-7.1648, 17.435)
  line L1520 (-17.6003, 5.9813) -> (-17.5782, 6.064)
  line L1521 (-17.5782, 6.064) -> (-17.5177, 6.1245)
  line L1522 (-17.5177, 6.1245) -> (-17.435, 6.1467)
  line L1523 (-17.435, 6.1467) -> (-17.3485, 6.1103)
  line L1524 (-17.3485, 6.1103) -> (-17.2918, 6.064)
  line L1525 (-17.2918, 6.064) -> (-17.2697, 5.9813)
  line L1526 (-17.2697, 5.9813) -> (-17.2918, 5.8987)
  line L1527 (-17.2918, 5.8987) -> (-17.3523, 5.8382)
  line L1528 (-17.3523, 5.8382) -> (-17.4331, 5.8179)
  line L1529 (-17.4331, 5.8179) -> (-17.5177, 5.8382)
  line L1530 (-17.5177, 5.8382) -> (-17.5782, 5.8987)
  line L1531 (-17.5782, 5.8987) -> (-17.6003, 5.9813)
  line L1532 (-17.6003, 0.8908) -> (-17.5782, 0.9735)
  line L1533 (-17.5782, 0.9735) -> (-17.5177, 1.034)
  line L1534 (-17.5177, 1.034) -> (-17.435, 1.0562)
  line L1535 (-17.435, 1.0562) -> (-17.3555, 1.0459)
  line L1536 (-17.3555, 1.0459) -> (-17.2918, 0.9735)
  line L1537 (-17.2918, 0.9735) -> (-17.2697, 0.8908)
  line L1538 (-17.2697, 0.8908) -> (-17.2918, 0.8082)
  line L1539 (-17.2918, 0.8082) -> (-17.3523, 0.7476)
  line L1540 (-17.435, 0.7255) -> (-17.5177, 0.7476)
  line L1541 (-17.5177, 0.7476) -> (-17.5782, 0.8082)
  line L1542 (-17.5782, 0.8082) -> (-17.6003, 0.8908)
  line L1543 (-14.4188, -4.4542) -> (-14.3966, -4.3715)
  line L1544 (-14.3966, -4.3715) -> (-14.3361, -4.311)
  line L1545 (-14.3361, -4.311) -> (-14.2571, -4.2873)
  line L1546 (-14.2571, -4.2873) -> (-14.1708, -4.311)
  line L1547 (-14.1708, -4.311) -> (-14.1102, -4.3715)
  line L1548 (-14.1102, -4.3715) -> (-14.0881, -4.4542)
  line L1549 (-14.0881, -4.4542) -> (-14.1102, -4.5369)
  line L1550 (-14.1102, -4.5369) -> (-14.1749, -4.5941)
  line L1551 (-14.1749, -4.5941) -> (-14.2534, -4.6195)
  line L1552 (-14.2534, -4.6195) -> (-14.3361, -4.5974)
  line L1553 (-14.3361, -4.5974) -> (-14.3966, -4.5369)
  line L1554 (-14.3966, -4.5369) -> (-14.4188, -4.4542)
  line L1555 (-17.4731, -10.5628) -> (-17.4509, -10.4801)
  line L1556 (-17.4509, -10.4801) -> (-17.3904, -10.4196)
  line L1557 (-17.3188, -10.3864) -> (-17.2251, -10.4196)
  line L1558 (-17.2251, -10.4196) -> (-17.1645, -10.4801)
  line L1559 (-17.1645, -10.4801) -> (-17.1424, -10.5628)
  line L1560 (-17.1424, -10.5628) -> (-17.1619, -10.6555)
  line L1561 (-17.1619, -10.6555) -> (-17.2251, -10.706)
  line L1562 (-17.2251, -10.706) -> (-17.3077, -10.7282)
  line L1563 (-17.3077, -10.7282) -> (-17.3904, -10.706)
  line L1564 (-17.3904, -10.706) -> (-17.4509, -10.6455)
  line L1565 (-17.4509, -10.6455) -> (-17.4731, -10.5628)
  line L1566 (-14.546, -12.599) -> (-14.5239, -12.5163)
  line L1567 (-14.5239, -12.5163) -> (-14.4473, -12.4601)
  line L1568 (-14.4473, -12.4601) -> (-14.3807, -12.4337)
  line L1569 (-14.3807, -12.4337) -> (-14.298, -12.4558)
  line L1570 (-14.298, -12.4558) -> (-14.2375, -12.5163)
  line L1571 (-14.2375, -12.5163) -> (-14.2154, -12.599)
  line L1572 (-14.2154, -12.599) -> (-14.2387, -12.6772)
  line L1573 (-14.2387, -12.6772) -> (-14.298, -12.7422)
  line L1574 (-14.298, -12.7422) -> (-14.3807, -12.7644)
  line L1575 (-14.3807, -12.7644) -> (-14.4634, -12.7422)
  line L1576 (-14.4634, -12.7422) -> (-14.5239, -12.6817)
  line L1577 (-14.5239, -12.6817) -> (-14.546, -12.599)
  line L1578 (-15.8187, -6.9995) -> (-15.7965, -6.9168)
  line L1579 (-15.7965, -6.9168) -> (-15.736, -6.8563)
  line L1580 (-15.736, -6.8563) -> (-15.6591, -6.8283)
  line L1581 (-15.6591, -6.8283) -> (-15.5706, -6.8563)
  line L1582 (-15.5706, -6.8563) -> (-15.5101, -6.9168)
  line L1583 (-15.5101, -6.9168) -> (-15.488, -6.9995)
  line L1584 (-15.488, -6.9995) -> (-15.5101, -7.0821)
  line L1585 (-15.5101, -7.0821) -> (-15.5671, -7.1253)
  line L1586 (-15.5671, -7.1253) -> (-15.6533, -7.1648)
  line L1587 (-15.6533, -7.1648) -> (-15.736, -7.1426)
  line L1588 (-15.736, -7.1426) -> (-15.7965, -7.0821)
  line L1589 (-15.7965, -7.0821) -> (-15.8187, -6.9995)
  line L1590 (-14.546, -10.8173) -> (-14.5239, -10.7347)
  line L1591 (-14.5239, -10.7347) -> (-14.4448, -10.6791)
  line L1592 (-14.4448, -10.6791) -> (-14.3807, -10.652)
  line L1593 (-14.3807, -10.652) -> (-14.298, -10.6741)
  line L1594 (-14.298, -10.6741) -> (-14.2375, -10.7347)
  line L1595 (-14.2375, -10.7347) -> (-14.2154, -10.8173)
  line L1596 (-14.2154, -10.8173) -> (-14.2362, -10.9047)
  line L1597 (-14.2362, -10.9047) -> (-14.298, -10.9605)
  line L1598 (-14.298, -10.9605) -> (-14.3807, -10.9827)
  line L1599 (-14.3807, -10.9827) -> (-14.4634, -10.9605)
  line L1600 (-14.4634, -10.9605) -> (-14.5239, -10.9)
  line L1601 (-14.5239, -10.9) -> (-14.546, -10.8173)
  line L1602 (-17.0913, -12.09) -> (-17.0691, -12.0073)
  line L1603 (-17.0691, -12.0073) -> (-17.0086, -11.9468)
  line L1604 (-16.9259, -11.9246) -> (-16.8433, -11.9468)
  line L1605 (-16.8433, -11.9468) -> (-16.7828, -12.0073)
  line L1606 (-16.7828, -12.0073) -> (-16.7606, -12.09)
  line L1607 (-16.7606, -12.09) -> (-16.7823, -12.1743)
  line L1608 (-16.7823, -12.1743) -> (-16.8433, -12.2332)
  line L1609 (-16.8433, -12.2332) -> (-16.9259, -12.2553)
  line L1610 (-16.9259, -12.2553) -> (-17.0086, -12.2332)
  line L1611 (-17.0086, -12.2332) -> (-17.0691, -12.1726)
  line L1612 (-17.0691, -12.1726) -> (-17.0913, -12.09)
  line L1613 (-17.3458, -13.6171) -> (-17.3237, -13.5344)
  line L1614 (-17.3237, -13.5344) -> (-17.2631, -13.4739)
  line L1615 (-17.1805, -13.4518) -> (-17.0978, -13.4739)
  line L1616 (-17.0978, -13.4739) -> (-17.0373, -13.5344)
  line L1617 (-17.0373, -13.5344) -> (-17.0151, -13.6171)
  line L1618 (-17.0151, -13.6171) -> (-17.0388, -13.694)
  line L1619 (-17.0388, -13.694) -> (-17.0978, -13.7603)
  line L1620 (-17.0978, -13.7603) -> (-17.1805, -13.7825)
  line L1621 (-17.1805, -13.7825) -> (-17.2631, -13.7603)
  line L1622 (-17.2631, -13.7603) -> (-17.3237, -13.6998)
  line L1623 (-17.3237, -13.6998) -> (-17.3458, -13.6171)
  line L1624 (-11.2372, -15.3988) -> (-11.215, -15.3161)
  line L1625 (-11.215, -15.3161) -> (-11.1593, -15.2543)
  line L1626 (-11.1593, -15.2543) -> (-11.0719, -15.2335)
  line L1627 (-11.0719, -15.2335) -> (-10.9892, -15.2556)
  line L1628 (-10.9892, -15.2556) -> (-10.9287, -15.3161)
  line L1629 (-10.9287, -15.3161) -> (-10.9065, -15.3988)
  line L1630 (-10.9287, -15.4815) -> (-10.9892, -15.542)
  line L1631 (-10.9892, -15.542) -> (-11.0719, -15.5641)
  line L1632 (-11.0719, -15.5641) -> (-11.1545, -15.542)
  line L1633 (-11.1545, -15.542) -> (-11.215, -15.4815)
  line L1634 (-11.215, -15.4815) -> (-11.2372, -15.3988)
  line L1635 (-11.2372, -17.435) -> (-11.215, -17.3523)
  line L1636 (-11.215, -17.3523) -> (-11.1621, -17.2898)
  line L1637 (-11.1621, -17.2898) -> (-11.0719, -17.2697)
  line L1638 (-11.0719, -17.2697) -> (-10.9892, -17.2918)
  line L1639 (-10.9892, -17.2918) -> (-10.9287, -17.3523)
  line L1640 (-10.9287, -17.3523) -> (-10.8944, -17.4471)
  line L1641 (-10.9287, -17.5177) -> (-10.9892, -17.5782)
  line L1642 (-10.9892, -17.5782) -> (-11.0719, -17.6003)
  line L1643 (-11.0719, -17.6003) -> (-11.1545, -17.5782)
  line L1644 (-11.1545, -17.5782) -> (-11.215, -17.5177)
  line L1645 (-11.215, -17.5177) -> (-11.2372, -17.435)
  line L1646 (-8.9465, -17.435) -> (-8.9243, -17.3523)
  line L1647 (-8.8832, -17.2866) -> (-8.7811, -17.2697)
  line L1648 (-8.7811, -17.2697) -> (-8.6985, -17.2918)
  line L1649 (-8.6985, -17.2918) -> (-8.6379, -17.3523)
  line L1650 (-8.6379, -17.3523) -> (-8.61, -17.4408)
  line L1651 (-8.61, -17.4408) -> (-8.6379, -17.5177)
  line L1652 (-8.6379, -17.5177) -> (-8.6985, -17.5782)
  line L1653 (-8.6985, -17.5782) -> (-8.7811, -17.6003)
  line L1654 (-8.7811, -17.6003) -> (-8.8638, -17.5782)
  line L1655 (-8.8638, -17.5782) -> (-8.9243, -17.5177)
  line L1656 (-8.9243, -17.5177) -> (-8.9465, -17.435)
  line L1657 (-6.6557, -17.435) -> (-6.6167, -17.3478)
  line L1658 (-6.6167, -17.3478) -> (-6.5731, -17.2918)
  line L1659 (-6.5731, -17.2918) -> (-6.4904, -17.2697)
  line L1660 (-6.4904, -17.2697) -> (-6.4077, -17.2918)
  line L1661 (-6.4077, -17.2918) -> (-6.3472, -17.3523)
  line L1662 (-6.3472, -17.3523) -> (-6.3256, -17.4345)
  line L1663 (-6.3256, -17.4345) -> (-6.3472, -17.5177)
  line L1664 (-6.3472, -17.5177) -> (-6.4077, -17.5782)
  line L1665 (-6.4077, -17.5782) -> (-6.4904, -17.6003)
  line L1666 (-6.4904, -17.6003) -> (-6.5731, -17.5782)
  line L1667 (-6.5731, -17.5782) -> (-6.6336, -17.5177)
  line L1668 (-6.6336, -17.5177) -> (-6.6557, -17.435)
  line L1669 (-0.0381, -17.435) -> (-0.0331, -17.3569)
  line L1670 (-0.0331, -17.3569) -> (0.0446, -17.2918)
  line L1671 (0.0446, -17.2918) -> (0.1273, -17.2697)
  line L1672 (0.1273, -17.2697) -> (0.2099, -17.2918)
  line L1673 (0.2099, -17.2918) -> (0.2863, -17.3566)
  line L1674 (0.2863, -17.3566) -> (0.2926, -17.435)
  line L1675 (0.2926, -17.435) -> (0.2705, -17.5177)
  line L1676 (0.2705, -17.5177) -> (0.2099, -17.5782)
  line L1677 (0.2099, -17.5782) -> (0.1273, -17.6003)
  line L1678 (0.1273, -17.6003) -> (0.0446, -17.5782)
  line L1679 (0.0446, -17.5782) -> (-0.0159, -17.5177)
  line L1680 (-0.0159, -17.5177) -> (-0.0381, -17.435)
  line L1681 (5.813, -15.6563) -> (5.8382, -15.5706)
  line L1682 (5.8382, -15.5706) -> (5.8987, -15.5101)
  line L1683 (5.8987, -15.5101) -> (5.9813, -15.488)
  line L1684 (5.9813, -15.488) -> (6.064, -15.5101)
  line L1685 (6.064, -15.5101) -> (6.1127, -15.5675)
  line L1686 (6.1127, -15.5675) -> (6.1467, -15.6533)
  line L1687 (6.1467, -15.6533) -> (6.1245, -15.736)
  line L1688 (6.1245, -15.736) -> (6.064, -15.7965)
  line L1689 (6.064, -15.7965) -> (5.9813, -15.8187)
  line L1690 (5.9813, -15.8187) -> (5.8987, -15.7965)
  line L1691 (5.8987, -15.7965) -> (5.8382, -15.736)
  line L1692 (5.8382, -15.736) -> (5.813, -15.6563)
  line L1693 (8.8568, -14.9033) -> (8.8925, -14.8071)
  line L1694 (8.8925, -14.8071) -> (8.953, -14.7466)
  line L1695 (8.953, -14.7466) -> (9.0357, -14.7244)
  line L1696 (9.0357, -14.7244) -> (9.1329, -14.7427)
  line L1697 (9.1329, -14.7427) -> (9.1788, -14.8071)
  line L1698 (9.1788, -14.8071) -> (9.201, -14.8897)
  line L1699 (9.201, -14.8897) -> (9.1788, -14.9724)
  line L1700 (9.1788, -14.9724) -> (9.1183, -15.0329)
  line L1701 (9.1183, -15.0329) -> (9.0357, -15.0551)
  line L1702 (9.0357, -15.0551) -> (8.953, -15.0329)
  line L1703 (8.953, -15.0329) -> (8.8925, -14.9724)
  line L1704 (11.6701, -14.8897) -> (11.6922, -14.8071)
  line L1705 (11.6922, -14.8071) -> (11.7528, -14.7466)
  line L1706 (11.7528, -14.7466) -> (11.8354, -14.7244)
  line L1707 (11.8354, -14.7244) -> (11.9183, -14.7465)
  line L1708 (11.9183, -14.7465) -> (11.9786, -14.8071)
  line L1709 (11.9786, -14.8071) -> (12.0008, -14.8897)
  line L1710 (12.0008, -14.8897) -> (11.9786, -14.9724)
  line L1711 (11.9786, -14.9724) -> (11.9181, -15.0329)
  line L1712 (11.9181, -15.0329) -> (11.8354, -15.0551)
  line L1713 (11.8354, -15.0551) -> (11.7528, -15.0329)
  line L1714 (11.7528, -15.0329) -> (11.6975, -14.9527)
  line L1715 (11.6975, -14.9527) -> (11.6701, -14.8897)
  line L1716 (13.4518, -15.9078) -> (13.4739, -15.8252)
  line L1717 (13.4739, -15.8252) -> (13.5344, -15.7647)
  line L1718 (13.5344, -15.7647) -> (13.6171, -15.7425)
  line L1719 (13.6171, -15.7425) -> (13.6922, -15.7667)
  line L1720 (13.6922, -15.7667) -> (13.7603, -15.8252)
  line L1721 (13.7603, -15.8252) -> (13.7825, -15.9078)
  line L1722 (13.7825, -15.9078) -> (13.7603, -15.9905)
  line L1723 (13.7603, -15.9905) -> (13.6998, -16.051)
  line L1724 (13.6998, -16.051) -> (13.6171, -16.0732)
  line L1725 (13.6171, -16.0732) -> (13.5344, -16.051)
  line L1726 (13.5344, -16.051) -> (13.4739, -15.9905)
  line L1727 (14.9789, -17.3077) -> (15.0011, -17.2251)
  line L1728 (15.0011, -17.2251) -> (15.0616, -17.1645)
  line L1729 (15.0616, -17.1645) -> (15.1443, -17.1424)
  line L1730 (15.1443, -17.1424) -> (15.2134, -17.1682)
  line L1731 (15.2134, -17.1682) -> (15.2875, -17.2251)
  line L1732 (15.2875, -17.2251) -> (15.3096, -17.3077)
  line L1733 (15.3096, -17.3077) -> (15.2875, -17.3904)
  line L1734 (15.2875, -17.3904) -> (15.2269, -17.4509)
  line L1735 (15.2269, -17.4509) -> (15.1443, -17.4731)
  line L1736 (15.1443, -17.4731) -> (15.0616, -17.4509)
  line L1737 (15.0616, -17.4509) -> (15.0011, -17.3904)
  line L1738 (17.2918, -14.6798) -> (17.3523, -14.6193)
  line L1739 (17.3523, -14.6193) -> (17.435, -14.5971)
  line L1740 (17.5177, -14.6193) -> (17.5782, -14.6798)
  line L1741 (17.5782, -14.6798) -> (17.6003, -14.7625)
  line L1742 (17.6003, -14.7625) -> (17.5782, -14.8452)
  line L1743 (17.5782, -14.8452) -> (17.5177, -14.9057)
  line L1744 (17.5177, -14.9057) -> (17.435, -14.9278)
  line L1745 (17.435, -14.9278) -> (17.3523, -14.9057)
  line L1746 (17.3523, -14.9057) -> (17.2949, -14.8338)
  line L1747 (17.2949, -14.8338) -> (17.2697, -14.7625)
  line L1748 (15.488, -13.3626) -> (15.5101, -13.2799)
  line L1749 (15.5101, -13.2799) -> (15.5706, -13.2194)
  line L1750 (15.5706, -13.2194) -> (15.6533, -13.1972)
  line L1751 (15.736, -13.2194) -> (15.7965, -13.2799)
  line L1752 (15.7965, -13.2799) -> (15.8187, -13.3626)
  line L1753 (15.8187, -13.3626) -> (15.7965, -13.4453)
  line L1754 (15.7965, -13.4453) -> (15.736, -13.5058)
  line L1755 (15.736, -13.5058) -> (15.6533, -13.5279)
  line L1756 (15.6533, -13.5279) -> (15.5706, -13.5058)
  line L1757 (15.5706, -13.5058) -> (15.5119, -13.4386)
  line L1758 (15.5119, -13.4386) -> (15.488, -13.3626)
  line L1759 (14.9789, -11.5809) -> (15.0011, -11.4982)
  line L1760 (15.0011, -11.4982) -> (15.0616, -11.4377)
  line L1761 (17.2697, 0.8908) -> (17.2918, 0.9735)
  line L1762 (17.2918, 0.9735) -> (17.3555, 1.0459)
  line L1763 (17.3555, 1.0459) -> (17.435, 1.0562)
  line L1764 (17.435, 1.0562) -> (17.5177, 1.034)
  line L1765 (17.5177, 1.034) -> (17.5782, 0.9735)
  line L1766 (17.5782, 0.9735) -> (17.6003, 0.8908)
  line L1767 (17.6003, 0.8908) -> (17.5782, 0.8082)
  line L1768 (17.5782, 0.8082) -> (17.5177, 0.7476)
  line L1769 (17.5177, 0.7476) -> (17.435, 0.7255)
  line L1770 (17.3523, 0.7476) -> (17.2918, 0.8082)
  line L1771 (17.2918, 0.8082) -> (17.2697, 0.8908)
  line L1772 (17.2697, 3.6906) -> (17.2918, 3.7733)
  line L1773 (17.3523, 3.8338) -> (17.435, 3.856)
  line L1774 (17.435, 3.856) -> (17.5177, 3.8338)
  line L1775 (17.5177, 3.8338) -> (17.5782, 3.7733)
  line L1776 (17.5782, 3.7733) -> (17.6003, 3.6906)
  line L1777 (17.6003, 3.6906) -> (17.5782, 3.6079)
  line L1778 (17.5782, 3.6079) -> (17.5177, 3.5474)
  line L1779 (17.5177, 3.5474) -> (17.4268, 3.5335)
  line L1780 (17.4268, 3.5335) -> (17.3523, 3.5474)
  line L1781 (17.3523, 3.5474) -> (17.2918, 3.6079)
  line L1782 (17.2918, 3.6079) -> (17.2697, 3.6906)
  line L1783 (17.2697, 9.2902) -> (17.2873, 9.3896)
  line L1784 (17.3523, 9.4334) -> (17.435, 9.4555)
  line L1785 (17.435, 9.4555) -> (17.5177, 9.4334)
  line L1786 (17.5177, 9.4334) -> (17.5782, 9.3729)
  line L1787 (17.5782, 9.3729) -> (17.6003, 9.2902)
  line L1788 (17.6003, 9.2902) -> (17.5782, 9.2075)
  line L1789 (17.5782, 9.2075) -> (17.5177, 9.147)
  line L1790 (17.5177, 9.147) -> (17.4422, 9.1176)
  line L1791 (17.4422, 9.1176) -> (17.3523, 9.147)
  line L1792 (17.3523, 9.147) -> (17.2918, 9.2075)
  line L1793 (17.2918, 9.2075) -> (17.2697, 9.2902)
  line L1794 (17.2697, 11.5809) -> (17.2905, 11.6686)
  line L1795 (17.2905, 11.6686) -> (17.3523, 11.7241)
  line L1796 (17.3523, 11.7241) -> (17.435, 11.7463)
  line L1797 (17.435, 11.7463) -> (17.5177, 11.7241)
  line L1798 (17.5177, 11.7241) -> (17.5782, 11.6636)
  line L1799 (17.5782, 11.6636) -> (17.6003, 11.5809)
  line L1800 (17.6003, 11.5809) -> (17.5782, 11.4982)
  line L1801 (17.5782, 11.4982) -> (17.5177, 11.4377)
  line L1802 (17.4485, 11.4021) -> (17.3523, 11.4377)
  line L1803 (17.3523, 11.4377) -> (17.2918, 11.4982)
  line L1804 (17.2918, 11.4982) -> (17.2697, 11.5809)
  line L1805 (17.3458, 12.8535) -> (17.3237, 12.7709)
  line L1806 (17.3237, 12.7709) -> (17.2631, 12.7103)
  line L1807 (17.1805, 12.6882) -> (17.0978, 12.7103)
  line L1808 (17.0978, 12.7103) -> (17.0373, 12.7709)
  line L1809 (17.0373, 12.7709) -> (17.0151, 12.8535)
  line L1810 (13.983, 17.5177) -> (14.0435, 17.5782)
  line L1811 (14.0435, 17.5782) -> (14.1262, 17.6003)
  line L1812 (14.1262, 17.6003) -> (14.2088, 17.5782)
  line L1813 (14.2088, 17.5782) -> (14.2694, 17.5177)
  line L1814 (14.2694, 17.5177) -> (14.2915, 17.435)
  line L1815 (14.2915, 17.435) -> (14.2694, 17.3523)
  line L1816 (14.2694, 17.3523) -> (14.2007, 17.294)
  line L1817 (14.2007, 17.294) -> (14.1262, 17.2697)
  line L1818 (14.1262, 17.2697) -> (14.0435, 17.2918)
  line L1819 (14.0435, 17.2918) -> (13.983, 17.3523)
  line L1820 (13.983, 17.3523) -> (13.9608, 17.435)
  line L1821 (12.7103, 17.5177) -> (12.7709, 17.5782)
  line L1822 (12.7709, 17.5782) -> (12.8535, 17.6003)
  line L1823 (12.8535, 17.6003) -> (12.9362, 17.5782)
  line L1824 (12.9362, 17.5782) -> (12.9967, 17.5177)
  line L1825 (12.9967, 17.5177) -> (13.0189, 17.435)
  line L1826 (13.0189, 17.435) -> (12.9967, 17.3523)
  line L1827 (12.9967, 17.3523) -> (12.9347, 17.2922)
  line L1828 (12.9347, 17.2922) -> (12.8535, 17.2697)
  line L1829 (12.8535, 17.2697) -> (12.7709, 17.2918)
  line L1830 (12.7709, 17.2918) -> (12.7103, 17.3523)
  line L1831 (12.7103, 17.3523) -> (12.6882, 17.435)
  line L1832 (10.6741, 17.5177) -> (10.7347, 17.5782)
  line L1833 (10.7347, 17.5782) -> (10.8173, 17.6003)
  line L1834 (10.8173, 17.6003) -> (10.9, 17.5782)
  line L1835 (10.9, 17.5782) -> (10.9605, 17.5177)
  line L1836 (10.9605, 17.5177) -> (10.9827, 17.435)
  line L1837 (10.9827, 17.435) -> (10.9605, 17.3523)
  line L1838 (10.9605, 17.3523) -> (10.9089, 17.2894)
  line L1839 (10.9089, 17.2894) -> (10.8173, 17.2697)
  line L1840 (10.8173, 17.2697) -> (10.7347, 17.2918)
  line L1841 (10.7347, 17.2918) -> (10.6741, 17.3523)
  line L1842 (10.6741, 17.3523) -> (10.6406, 17.4464)
  line L1843 (15.997, 11.8354) -> (16.0192, 11.9181)
  line L1844 (16.0797, 11.9786) -> (16.1624, 12.0008)
  line L1845 (16.245, 11.9786) -> (16.3056, 11.9181)
  line L1846 (16.3277, 11.8354) -> (16.3056, 11.7528)
  line L1847 (16.3056, 11.7528) -> (16.245, 11.6922)
  line L1848 (16.1624, 11.6701) -> (16.0797, 11.6922)
  line L1849 (6.3168, 14.2617) -> (6.3472, 14.3361)
  line L1850 (6.3472, 14.3361) -> (6.4077, 14.3966)
  line L1851 (6.4077, 14.3966) -> (6.4904, 14.4188)
  line L1852 (6.4904, 14.4188) -> (6.5731, 14.3966)